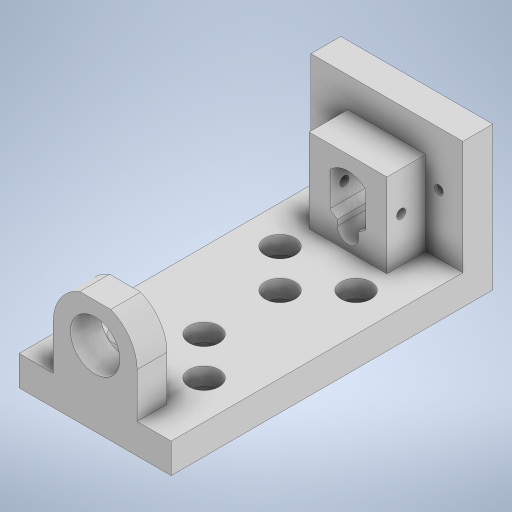
# Autodesk Inventor part: Actuator Mount
Saved by Autodesk Inventor 2024 (Build 280153000, 153)
## iProperties
Company: University of California - Davis
Created: 2024-11-19
Part Number: Actuator Mount
Material: Generic
Document SubType Name: Modeling
Designer: Scott J. Bricker
Density: 1 g/cm^3
Appearance: Default
Project: Firgelli Motorized Linear Stage
Engineer: Scott J. Bricker
Author: Scott J. Bricker
Title: Actuator Mount
Subject: Firgelli Motorized Linear Stage
Revision Number: 1.1 P3
Autodesk Inventor part; units mm, degrees
ref_plane "YZ Plane" through (0, 0, 0) normal (1, 0, 0) x (0, 1, 0)
ref_plane "XZ Plane" through (0, 0, 0) normal (0, 1, 0) x (-1, 0, 0)
sketch "Sketch1" plane through (0, 0, 0) normal (0, 0, 1) x (1, 0, 0)
  line L0 (0, 0) -> (0, 4)
  line L1 (0, 4) -> (0, 10)
  line L2 (0, 10) -> (0, 38)
  line L3 (0, 38) -> (0, 48)
  line L4 (0, 0) -> (50.8, 0)
  line L5 (50.8, 0) -> (50.8, 48)
  line L6 (50.8, 48) -> (0, 48)
  dimension "d1" = 4
  dimension "d2" = 6
  dimension "d3" = 28
  dimension "d4" = 10
  dimension "d5" = 50.8
  constraints: 14 end point, 3 point on line, 2 perpendicular, 1 horizontal, 1 vertical
  measures "d1" distance of L0.start L0.end
  measures "d2" distance of L0.end L1.end
  measures "d3" distance of L1.end L2.end
  measures "d4" distance of L2.end L3.end
  measures "d5" distance of L0.start L4.end
extrude "Extrusion1" add sketch "Sketch1" along normal blind 10
sketch "Sketch2" plane through (0, 0, 10) normal (0, 0, 1) x (1, 0, 0)
  line L0 (50.8, 48) -> (0, 48) projected
  line L1 (0, 48) -> (0, 0) projected
  line L2 (0, 0) -> (50.8, 0) projected
  line L3 (50.8, 0) -> (50.8, 48) projected
  line L4 (0, 0) -> (50.8, 0)
  line L5 (50.8, 0) -> (50.8, 10)
  line L6 (50.8, 10) -> (0, 10)
  line L7 (0, 10) -> (0, 0)
  point P0 (0, 10)
  dimension "d8" = 10
  constraints: 8 end point, 2 parallel, 1 horizontal, 1 perpendicular, 1 point on line
  measures "d8" distance between parallel lines of L6 L2
extrude "Extrusion2" add sketch "Sketch2" along normal blind 87.5 contours L3 L2 L1 L6
sketch "Sketch3" plane through (0, 0, 10) normal (0, 0, 1) x (1, 0, 0)
  line L0 (0, 10) -> (50.8, 10) projected
  line L1 (50.8, 10) -> (50.8, 48) projected
  line L2 (50.8, 48) -> (0, 48) projected
  line L3 (0, 48) -> (0, 10) projected
  line L4 (12.4, 12) -> (38.4, 12)
  line L5 (38.4, 12) -> (38.4, 38)
  line L6 (38.4, 38) -> (12.4, 38)
  line L7 (12.4, 38) -> (12.4, 12)
  line L8 (50.8, 10) -> (0, 10) projected
  line L9 (38.4, 10) -> (12.4, 10)
  line L10 (12.4, 12) -> (38.4, 12)
  line L11 (38.4, 12) -> (38.4, 10)
  line L12 (38.4, 10) -> (12.4, 10)
  line L13 (12.4, 10) -> (12.4, 12)
  arc A0 (28.9, 20.1266) -> (21.9, 20.1266) centre (25.4, 25) ccw
  line L14 (19.4, 30.6624) -> (19.4, 19.3376)
  line L15 (31.4, 30.6624) -> (31.4, 19.3376)
  line L16 (23.3844, 17) -> (27.4156, 17)
  arc A1 (19.4, 19.3376) -> (23.3844, 17) centre (25.4, 25) ccw
  arc A2 (27.4156, 17) -> (31.4, 19.3376) centre (25.4, 25) ccw
  arc A3 (21.9, 18) -> (28.9, 18) centre (25.4, 18) ccw
  line L17 (21.9, 18) -> (28.9, 18)
  line L18 (28.9, 18) -> (28.9, 20.1266)
  line L19 (21.9, 20.1266) -> (21.9, 18)
  circle A4 centre (25.4, 25) radius 8.25
  point P0 (0, 0)
  point P1 (25.4, 10)
  point P2 (25.4, 12)
  point P3 (38.4, 25)
  point P4 (12.4, 25)
  point P5 (25.4, 38)
  point P6 (19.4, 25)
  point P7 (28.866, 17.5134)
  point P8 (21.934, 17.5134)
  dimension "d12" = 0
  dimension "d13" = 26
  dimension "d14" = 26
  dimension "d19" = 10
  dimension "d22" = 0
  dimension "d23" = 0
  dimension "d25" = 12
  dimension "d26" = 0
  dimension "d27" = 0
  dimension "d28" = 7
  dimension "d29" = 0
  dimension "d31" = 7
  dimension "d32" = 16.5
  constraints: 30 end point, 8 point on circle, 5 centre point, 5 midpoint, 5 parallel, 3 horizontal, 3 perpendicular, 2 coincident, 2 point on line
  measures "d12" horizontal distance of point (25.4, 10) point (25.4, 12)
  measures "d13" distance of L4.start L4.end
  measures "d14" distance of L4.end L5.end
  measures "d19" distance between parallel lines of L2 L6
  measures "d22" vertical distance of point (12.4, 25) A0.centre
  measures "d23" horizontal distance of point (25.4, 38) A0.centre
  measures "d25" diameter of A0
  measures "d26" distance edge to line of A0 L15
  measures "d27" distance edge to line of A0 L14
  measures "d28" diameter of A3
  measures "d29" horizontal distance of A0.centre A3.centre
  measures "d31" distance of A0.centre A3.centre
  measures "d32" diameter of A4
extrude "Extrusion3" add sketch "Sketch3" along normal blind 13 contours L13 L4 L11 L0 | L7 L6 L5 L4 | L15 A4 | L14 A4
ref_plane "Work Plane1" through (25.4, 10, 10) normal (1, 0, 0) x (0, 0, -1)
sketch "Sketch4" plane through (25.4, 10, 10) normal (1, 0, 0) x (0, 0, -1)
  line L0 (0, 20.6624) -> (0, 9.3376) projected
  line L1 (0, 20.6624) -> (-13, 20.6624) projected
  line L2 (-13, 9.3376) -> (-13, 20.6624) projected
  line L3 (0, 9.3376) -> (-13, 9.3376) projected
  circle A0 centre (-8.25, 15) radius 1.5
  point P0 (10, -10)
  point P1 (-13, 15)
  dimension "d34" = 0
  dimension "d35" = 8.25
  dimension "d36" = 3
  constraints: 1 centre point, 1 midpoint
  measures "d34" vertical distance of point (-13, 15) A0.centre
  measures "d35" distance from line of L0 A0.centre
  measures "d36" diameter of A0
extrude "Extrusion4" cut sketch "Sketch4" along normal mid plane 26 contours A0
sketch "Sketch5" plane through (0, 10, 97.5) normal (0, 1, 0) x (1, 0, 0)
  line L0 (12.4, 74.5) -> (12.4, 87.5) projected
  line L1 (0, 87.5) -> (12.4, 87.5) projected
  line L2 (0, 87.5) -> (0, 0) projected
  line L3 (50.8, 0) -> (0, 0) projected
  line L4 (50.8, 87.5) -> (50.8, 0) projected
  line L5 (38.4, 87.5) -> (50.8, 87.5) projected
  line L6 (38.4, 87.5) -> (38.4, 74.5) projected
  line L7 (38.4, 74.5) -> (12.4, 74.5) projected
  circle A0 centre (25.4, 51.8) radius 3.175
  line L8 (50.8, 87.5) -> (0, 87.5) projected
  circle A1 centre (12.7, 64.5) radius 3.175
  circle A2 centre (38.1, 64.5) radius 3.175
  line L9 (-10.8452, 39.1) -> (75.4395, 39.1)
  circle A3 centre (25.4, 26.4) radius 3.175
  circle A4 centre (12.7, 13.7) radius 3.175
  circle A5 centre (38.1, 13.7) radius 3.175
  point P0 (0, 97.5)
  point P1 (25.4, 0)
  dimension "d39" = 35.7
  dimension "d40" = 0
  dimension "d41" = 6.35
  dimension "d42" = 12.7
  dimension "d43" = 12.7
  dimension "d44" = 12.7
  dimension "d45" = 12.7
  dimension "d46" = 12.7
  dimension "d73" = 6.35
  dimension "d74" = 6.35
  constraints: 6 centre point, 3 symmetric about line, 2 end point, 1 horizontal, 1 midpoint, 3 other
  measures "d39" distance from line of L8 A0.centre
  measures "d40" horizontal distance of point (25.4, 0) A0.centre
  measures "d41" diameter of A0
  measures "d42" horizontal distance of A1.centre A0.centre
  measures "d43" distance from line of L9 A0.centre
  measures "d44" horizontal distance of A0.centre A1.centre
  measures "d45" horizontal distance of A2.centre A0.centre
  measures "d46" horizontal distance of A0.centre A2.centre
  measures "d73" diameter of A1
  measures "d74" diameter of A2
extrude "Extrusion5" cut sketch "Sketch5" against normal blind 26 contours A0 | A1 | A2 | A3 | A4 | A5
sketch "Sketch6" plane through (0, 0, 0) normal (0, 0, -1) x (-1, 0, 0)
  line L0 (-12.4, 10) -> (-12.4, 38) projected
  line L1 (-12.4, 38) -> (-38.4, 38) projected
  line L2 (-38.4, 38) -> (-38.4, 10) projected
  line L3 (-38.4, 10) -> (-50.8, 10) projected
  line L4 (-50.8, 10) -> (-50.8, 48) projected
  line L5 (-50.8, 48) -> (0, 48) projected
  line L6 (0, 48) -> (0, 10) projected
  line L7 (0, 10) -> (-12.4, 10) projected
  circle A0 centre (-42.8, 30) radius 1.42
  line L8 (-25.4, -18.8015) -> (-25.4, 63.6237)
  circle A1 centre (-8, 30) radius 1.42
  point P0 (0, 0)
  point P1 (-25.4, 48)
  dimension "d49" = 0
  dimension "d50" = 8
  dimension "d51" = 8
  dimension "d52" = 2.84
  constraints: 2 centre point, 2 end point, 1 midpoint, 1 symmetric about line, 1 vertical, 1 other
  measures "d49" distance from line of point (-25.4, 48) L8
  measures "d50" distance from line of L1 A0.centre
  measures "d51" distance from line of L4 A0.centre
  measures "d52" diameter of A0
extrude "Extrusion6" cut sketch "Sketch6" against normal blind 26 contours A0 | A1
sketch "Sketch7" plane through (0, 0, 97.5) normal (0, 0, 1) x (1, 0, 0)
  line L0 (0, 10) -> (0, 0) projected
  line L1 (0, 0) -> (50.8, 0) projected
  line L2 (50.8, 0) -> (50.8, 10) projected
  line L3 (50.8, 10) -> (0, 10) projected
  line L4 (12.4, 38) -> (12.4, 10) projected
  line L5 (38.4, 10) -> (12.4, 10) projected
  line L6 (38.4, 10) -> (38.4, 38) projected
  line L7 (38.4, 38) -> (12.4, 38) projected
  arc A0 (31.4, 30.6624) -> (19.4, 30.6624) centre (25.4, 25) ccw projected
  line L8 (31.4, 30.6624) -> (31.4, 19.3376) projected
  arc A1 (28.866, 17.5134) -> (31.4, 19.3376) centre (25.4, 25) ccw projected
  arc A2 (21.934, 17.5134) -> (28.866, 17.5134) centre (25.4, 18) ccw projected
  arc A3 (19.4, 19.3376) -> (21.934, 17.5134) centre (25.4, 25) ccw projected
  line L9 (19.4, 19.3376) -> (19.4, 30.6624) projected
  circle A4 centre (25.4, 25) radius 14
  circle A5 centre (25.4, 25) radius 8.25
  line L10 (11.4, 25) -> (11.4, 10)
  line L11 (39.4, 25) -> (39.4, 10)
  line L12 (0, 10) -> (50.8, 10)
  line L13 (50.8, 10) -> (50.8, 0)
  line L14 (50.8, 0) -> (0, 0)
  line L15 (0, 0) -> (0, 10)
  circle A6 centre (8, 30) radius 1.42 projected
  circle A7 centre (42.8, 30) radius 1.42 projected
  line L16 (12.4, 10) -> (12.4, 38) projected
  line L17 (12.4, 38) -> (38.4, 38) projected
  line L18 (38.4, 38) -> (38.4, 10) projected
  line L19 (38.4, 10) -> (50.8, 10) projected
  line L20 (50.8, 10) -> (50.8, 48) projected
  line L21 (50.8, 48) -> (0, 48) projected
  line L22 (0, 48) -> (0, 10) projected
  line L23 (0, 10) -> (12.4, 10) projected
  circle A8 centre (8, 30) radius 3
  circle A9 centre (42.8, 30) radius 3
  line L24 (12.4, 38) -> (38.4, 38)
  line L25 (38.4, 38) -> (38.4, 42.0795)
  line L26 (38.4, 42.0795) -> (12.4, 42.0795)
  line L27 (12.4, 42.0795) -> (12.4, 38)
  point P0 (30.5962, 38)
  point P1 (20.2038, 38)
  dimension "d55" = 28
  dimension "d56" = 16.5
  dimension "d57" = 6
  dimension "d58" = 6
  constraints: 20 end point, 4 centre point, 4 coincident, 4 parallel, 4 perpendicular, 2 horizontal, 2 point on circle, 2 point on line, 1 tangent
  measures "d55" diameter of A4
  measures "d56" diameter of A5
  measures "d57" diameter of A8
  measures "d58" diameter of A9
extrude "Extrusion7" add sketch "Sketch7" along normal blind 10 contours L3 L2 L1 L0 | L10 A4 L4 L3 | L4 A4 L6 L3 | A4 L4 | L6 A4 L11 L3 | L4 A4 L7 L6 | L6 A4 | A2 A5
sketch "Sketch8" plane through (0, 10, 10) normal (0, 1, 0) x (1, 0, 0)
  circle A0 centre (38.1, -73.8) radius 3.175 projected
  circle A1 centre (38.1, -23) radius 3.175 projected
  circle A2 centre (25.4, -61.1) radius 3.175 projected
  circle A3 centre (25.4, -35.7) radius 3.175 projected
  circle A4 centre (12.7, -23) radius 3.175 projected
  circle A5 centre (12.7, -73.8) radius 3.175 projected
  line L0 (12.4, -13) -> (12.4, 0) projected
  line L1 (0, 0) -> (12.4, 0) projected
  line L2 (0, 0) -> (0, -97.5) projected
  line L3 (11.4, -97.5) -> (0, -97.5) projected
  line L4 (11.4, -87.5) -> (11.4, -97.5) projected
  line L5 (39.4, -87.5) -> (11.4, -87.5) projected
  line L6 (39.4, -87.5) -> (39.4, -97.5) projected
  line L7 (50.8, -97.5) -> (39.4, -97.5) projected
  line L8 (50.8, 0) -> (50.8, -97.5) projected
  line L9 (38.4, 0) -> (50.8, 0) projected
  line L10 (38.4, 0) -> (38.4, -13) projected
  line L11 (38.4, -13) -> (12.4, -13) projected
  circle A6 centre (25.4, -35.7) radius 5
  circle A7 centre (12.7, -23) radius 5
  circle A8 centre (38.1, -23) radius 5
  circle A9 centre (25.4, -61.1) radius 5
  circle A10 centre (12.7, -73.8) radius 3.175 projected
  circle A11 centre (12.7, -73.8) radius 5
  circle A12 centre (38.1, -73.8) radius 5
  point P0 (0, 10)
  dimension "d61" = 10
  dimension "d62" = 10
  dimension "d63" = 10
  dimension "d64" = 10
  dimension "d65" = 10
  dimension "d66" = 10
  constraints: 6 centre point, 6 coincident
  measures "d61" diameter of A6
  measures "d62" diameter of A9
  measures "d63" diameter of A8
  measures "d64" diameter of A7
  measures "d65" diameter of A12
  measures "d66" diameter of A11
extrude "Extrusion8" cut sketch "Sketch8" against normal blind 6 contours A2 | A6 | A7 | A8 | A9 | A11 | A12
sketch "Sketch9" plane through (0, 0, 0) normal (0, 0, -1) x (-1, 0, 0)
  circle A0 centre (-8, 30) radius 1.42 projected
  circle A1 centre (-42.8, 30) radius 1.42 projected
  line L0 (-50.8, 48) -> (0, 48) projected
  line L1 (-50.8, 0) -> (-50.8, 48) projected
  line L2 (0, 0) -> (-50.8, 0) projected
  line L3 (0, 48) -> (0, 0) projected
  circle A2 centre (-42.8, 30) radius 5
  circle A3 centre (-8, 30) radius 5
  dimension "d69" = 10
  dimension "d70" = 10
  constraints: 2 centre point, 2 coincident
  measures "d69" diameter of A2
  measures "d70" diameter of A3
extrude "Extrusion9" cut sketch "Sketch9" against normal blind 5 contours A1 | A2 | A3
sketch "Sketch10" plane through (0, 0, 23) normal (0, 0, 1) x (1, 0, 0)
  line L0 (12.4, 38) -> (12.4, 10) projected
  line L1 (38.4, 10) -> (12.4, 10) projected
  line L2 (38.4, 10) -> (38.4, 38) projected
  line L3 (38.4, 38) -> (12.4, 38) projected
  arc A0 (31.4, 30.6624) -> (19.4, 30.6624) centre (25.4, 25) ccw projected
  line L4 (31.4, 30.6624) -> (31.4, 19.3376) projected
  arc A1 (28.866, 17.5134) -> (31.4, 19.3376) centre (25.4, 25) ccw projected
  arc A2 (21.934, 17.5134) -> (28.866, 17.5134) centre (25.4, 18) ccw projected
  arc A3 (19.4, 19.3376) -> (21.934, 17.5134) centre (25.4, 25) ccw projected
  line L5 (19.4, 19.3376) -> (19.4, 30.6624) projected
  circle A4 centre (25.4, 15.5) radius 3.5
  line L6 (21.9, 15.5) -> (28.9, 15.5)
  line L7 (28.9, 15.5) -> (28.9, 21)
  line L8 (28.9, 21) -> (21.9, 21)
  line L9 (21.9, 21) -> (21.9, 15.5)
  point P0 (0, 0)
  dimension "d75" = 7
  dimension "d76" = 5.5
  dimension "d77" = 0
  dimension "d78" = 7
  dimension "d79" = 5.5
  constraints: 8 end point, 2 parallel, 1 horizontal, 1 perpendicular, 3 other
  measures "d76" distance from line of L1 point (25.4, 15.5)
  measures "d77" horizontal distance of A2.centre point (25.4, 15.5)
  measures "d78" distance of L7.end L8.end
  measures "d79" distance from line of point (25.4, 15.5) L8
extrude "Extrusion10" cut sketch "Sketch10" against normal through all contours L7 A4 A2 A1 | A1 A2 A4 A3 L9 L8 L7 | A3 A2 A4 L9 | L6 A2 A4 | A4 L6 A2 | A4 A2 L6 | A2 L6 A4 | A2 L6
fillet "Fillet1" radius 2 7 edges at (25.4, 21, 10) (21.9, 19.2646, 10) (28.9, 19.2646, 10) (28.9, 18.25, 0) (21.9, 18.25, 0) (25.4, 12, 0) (25.4, 21, 0)
equation "\"d4\" = Thick_Wall"
equation "\"d5\" = Platform_Width"
equation "\"d6\" = Thick_Wall"
equation "\"d8\" = d1 + d2"
equation "\"d19\" = Thick_Wall"
equation "\"d41\" = Tabletop_Hole_Diameter"
equation "\"d42\" = d43"
equation "\"d43\" = 0.5 * Tabletop_Hole_Spacing"
equation "\"d44\" = d43"
equation "\"d45\" = d43"
equation "\"d46\" = d43"
equation "\"d73\" = d41"
equation "\"d74\" = d41"
equation "\"d57\" = Guide_Rod_Diameter"
equation "\"d58\" = Guide_Rod_Diameter"
equation "\"d59\" = Thick_Wall"
equation "\"d62\" = d61"
equation "\"d63\" = d61"
equation "\"d64\" = d61"
equation "\"d65\" = d61"
equation "\"d66\" = d61"
equation "\"d67\" = d2"
equation "\"d71\" = 0.5 * Thick_Wall"
equation "\"d78\" = d75"
equation "\"Platform_Width\" = 50.8"
equation "\"Platform_Length\" = 245"
equation "\"Guide_Hole_Offset\" = 13.51"
equation "\"Guide_Rod_Diameter\" = 6"
equation "\"Guide_Rod_Length\" = 304.8"
equation "\"Thin_Wall\" = 5"
equation "\"Thick_Wall\" = 10"
equation "\"Tabletop_Hole_Spacing\" = 25.4"
equation "\"Tabletop_Hole_Diameter\" = 6.35"
equation "\"Platform_Hole_Spacing\" = 25.4"
equation "\"Platform_Hole_Diameter\" = 6.35"
equation "\"d15\" = Thin_Wall"
equation "\"d17\" = d15"
equation "\"Actuator_Housing_W\" = 26"
equation "\"Sliding_Clearance\" = 2"
equation "\"Platform_GuideRod_OD\" = 16.5"
body "Solid1"
